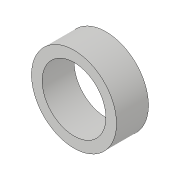
# Autodesk Inventor part: Pivot Rod Washer
Saved by Autodesk Inventor 2018.3 (Build 223284000, 284)
## iProperties
Created: 2019-05-29
Part Number: Pivot Rod Washer
Material: Generic
Document SubType Name: Modeling
Designer: aye06091
Mass: 0.0330809 g
Surface Area: 1.11064 cm^2
Volume: 0.0330809 cm^3
Density: 1 g/cm^3
Appearance: Default
Author: aye06091
Autodesk Inventor part; units mm, degrees
ref_plane "YZ Plane" through (0, 0, 0) normal (1, 0, 0) x (0, 1, 0)
ref_plane "XZ Plane" through (0, 0, 0) normal (0, 1, 0) x (-1, 0, 0)
ref_plane "XY Plane" through (0, 0, 0) normal (0, 0, 1) x (1, 0, 0)
sketch "Sketch1" plane through (0, 0, 0) normal (0, 0, 1) x (1, 0, 0)
  circle A0 centre (0, 0) radius 3.175
  dimension "d0" = 6.35
  constraints: 1 centre point, 1 coincident
  measures "d0" diameter of A0
extrude "Extrusion1" add sketch "Sketch1" against normal blind 2.3876
sketch "Sketch2" plane through (0, 0, 0) normal (0, 0, 1) x (1, 0, 0)
  circle A0 centre (0, 0) radius 3.175 projected
  circle A1 centre (0, 0) radius 2.3813
  dimension "d3" = 4.7625
  constraints: 1 centre point, 1 coincident
  measures "d3" diameter of A1
extrude "Extrusion2" cut sketch "Sketch2" against normal blind 3.175 contours A1
body "Solid1"
